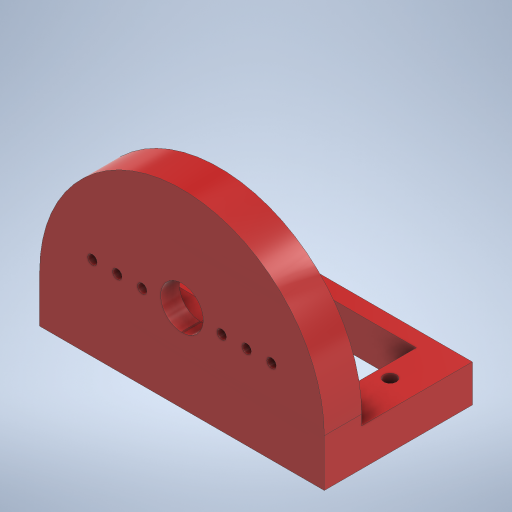
# Autodesk Inventor part: unions1s2lado2
Saved by Autodesk Inventor 2024.3 (Build 283343000, 343)
## iProperties
Created: 2025-08-12
Part Number: unions1s2lado2
Material: Generic
Document SubType Name: Modeling
Designer: jscme
Density: 1 g/cm^3
Appearance: Default
Author: jscme
Autodesk Inventor part; units mm, degrees
ref_plane "YZ Plane" through (0, 0, 0) normal (1, 0, 0) x (0, 1, 0)
ref_plane "XZ Plane" through (0, 0, 0) normal (0, 1, 0) x (-1, 0, 0)
ref_plane "XY Plane" through (0, 0, 0) normal (0, 0, 1) x (1, 0, 0)
sketch "Sketch1" plane through (0, 0, 0) normal (0, 1, 0) x (-1, 0, 0)
  line L0 (22.86, 8.89) -> (-22.86, 8.89)
  line L1 (-22.86, 8.89) -> (-22.86, -8.89)
  line L2 (-22.86, -8.89) -> (22.86, -8.89)
  line L3 (22.86, -8.89) -> (22.86, 8.89)
  point P0 (0, 0)
  point P1 (0, 0)
  point P2 (0, -8.89)
  point P3 (22.86, 0)
  dimension "d0" = 45.72
  dimension "d1" = 17.78
  constraints: 8 end point, 2 midpoint, 2 parallel, 1 coincident, 1 horizontal, 1 horizontal alignment, 1 perpendicular, 1 vertical alignment
  measures "d0" distance of L1.end L2.end
  measures "d1" distance of L0.end L1.end
extrude "Extrusion1" add sketch "Sketch1" along normal blind 6
sketch "Sketch2" plane through (0, 6, 0) normal (0, 1, 0) x (1, 0, 0)
  line L0 (-7.7264, -6.35) -> (16.4036, -6.35)
  line L1 (16.4036, -6.35) -> (16.4036, 6.35)
  line L2 (16.4036, 6.35) -> (-7.7264, 6.35)
  line L3 (-7.7264, 6.35) -> (-7.7264, -6.35)
  circle A0 centre (-9.86, 0) radius 1.016
  circle A1 centre (18.5372, 0) radius 1.016
  line L4 (22.86, -8.89) -> (22.86, 8.89) projected
  line L5 (-22.86, 8.89) -> (-22.86, -8.89) projected
  point P0 (4.3386, 0)
  point P1 (4.3386, 0)
  point P2 (-7.7264, 0)
  point P3 (4.3386, 6.35)
  point P4 (-22.86, 0)
  dimension "d4" = 24.13
  dimension "d5" = 12.7
  dimension "d6" = 2.032
  dimension "d7" = 2.032
  dimension "d8" = 2.1336
  dimension "d9" = 2.1336
  dimension "d31" = 13
  constraints: 8 end point, 3 horizontal alignment, 3 midpoint, 2 centre point, 2 coincident, 2 parallel, 1 horizontal, 1 perpendicular, 1 vertical alignment
  measures "d4" distance of L1.end L2.end
  measures "d5" distance of L2.end L0.start
  measures "d6" diameter of A0
  measures "d7" diameter of A1
  measures "d8" distance from line of L3 A0.centre
  measures "d9" distance from line of L1 A1.centre
  measures "d31" distance of point (-22.86, 0) A0.centre
extrude "Extrusion2" cut sketch "Sketch2" against normal through all
sketch "Sketch3" plane through (-22.86, 0, 8.89) normal (0, 0, 1) x (1, 0, 0)
  line L0 (45.72, 0) -> (0, 0) projected
  line L1 (0, 0) -> (0, 7.62)
  line L2 (45.72, 0) -> (45.72, 7.62)
  arc A0 (45.72, 7.62) -> (0, 7.62) centre (22.86, 7.62) ccw
  point P0 (22.86, 0)
  dimension "d12" = 7.62
  dimension "d13" = 7.62
  constraints: 4 end point, 2 point on circle, 2 vertical, 1 centre point, 1 tangent
  measures "d12" distance of L0.end L1.end
  measures "d13" distance of L0.start L2.end
extrude "Extrusion3" add sketch "Sketch3" along normal blind 6
sketch "Sketch4" plane through (-22.86, 0, 8.89) normal (0, 0, -1) x (-1, 0, 0)
  arc A0 (0, 7.62) -> (-45.72, 7.62) centre (-22.86, 7.62) ccw projected
  circle A1 centre (-22.86, 13.97) radius 3.429
  line L0 (-22.86, 17.399) -> (-37.8169, 16.12)
  line L1 (-22.86, 10.541) -> (-37.8686, 10.8324)
  arc A2 (-37.8169, 16.12) -> (-37.8686, 10.8324) centre (-37.5906, 13.4738) ccw
  arc A3 (-9.0266, 10.8096) -> (-8.8489, 16.2009) centre (-9.079, 13.5099) ccw
  line L2 (-22.86, 17.399) -> (-8.8489, 16.2009)
  line L3 (-22.86, 10.541) -> (-9.0266, 10.8096)
  point P0 (-22.86, 0)
  point P1 (-22.86, 30.48)
  point P2 (-22.86, 30.48)
  point P3 (-6.3797, 13.421)
  point P4 (-22.86, 30.48)
  point P5 (-23.4422, 17.3492)
  point P6 (-22.9931, 10.5436)
  point P7 (-22.7269, 10.5436)
  point P8 (-22.2778, 17.3492)
  dimension "d24" = 6
  dimension "d25" = 6.858
  dimension "d26" = 6
  dimension "d27" = 13.781
  dimension "d28" = 16.51
  constraints: 10 point on circle, 8 end point, 3 centre point, 3 tangent, 3 vertical alignment, 1 equal length
  measures "d24" angle of L1 L0
  measures "d25" diameter of A1
  measures "d26" angle of L2 L3
  measures "d27" horizontal distance of A3.centre A1.centre
  measures "d28" distance of point (-22.86, 30.48) A1.centre
extrude "Extrusion4" cut sketch "Sketch4" against normal blind 10 contours A1 L0 L2
extrude "Extrusion6" cut sketch "Sketch4" against normal blind 3 contours L1 A2 L0 A1 | A1 L2 A3 L3
sketch "Sketch5" plane through (-22.86, 0, 8.89) normal (0, 0, -1) x (-1, 0, 0)
  circle A0 centre (-37.2464, 13.4738) radius 0.75
  circle A1 centre (-33.2464, 13.4738) radius 0.75
  circle A2 centre (-29.2464, 13.4738) radius 0.75
  arc A3 (-37.8169, 16.12) -> (-37.8686, 10.8324) centre (-37.5906, 13.4738) ccw projected
  line L0 (-22.86, 20.4173) -> (-22.86, 7.5227)
  arc A4 (-23.4422, 17.3492) -> (-22.9931, 10.5436) centre (-22.86, 13.97) ccw projected
  arc A5 (-22.7269, 10.5436) -> (-22.2778, 17.3492) centre (-22.86, 13.97) ccw projected
  circle A6 centre (-12.4736, 13.4738) radius 0.75
  circle A7 centre (-8.4736, 13.4738) radius 0.75
  circle A8 centre (-16.4736, 13.4738) radius 0.75
  point P0 (-22.86, 0)
  point P1 (-40.2464, 13.4998)
  dimension "d32" = 1.5
  dimension "d36" = 1.5
  dimension "d37" = 1.5
  dimension "d44" = 3
  dimension "d49" = 4
  dimension "d50" = 4
  constraints: 6 centre point, 3 horizontal alignment, 3 symmetric about line, 2 end point, 1 coincident, 1 midpoint, 1 point on circle, 1 vertical, 3 other
  measures "d32" diameter of A0
  measures "d36" diameter of A1
  measures "d37" diameter of A2
  measures "d44" horizontal distance of point (-40.246, 13.5) A0.centre
  measures "d49" distance of A0.centre A1.centre
  measures "d50" distance of A1.centre A2.centre
extrude "Extrusion7" cut sketch "Sketch5" against normal through all
body "Solid1"
